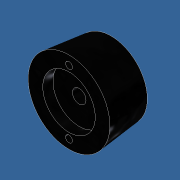
# Autodesk Inventor part: bouton
Saved by Autodesk Inventor 2015 SP2 (Build 190223200, 223)
## iProperties
Created: 2017-10-26
Part Number: bouton
Material: Générique
Document SubType Name: Modeling
Designer: Benoit.CURCHOD2
Density: 1 g/cm^3
Appearance: Noir
Author: Benoit.CURCHOD2
Autodesk Inventor part; units mm, degrees
ref_plane "YZ Plane" through (0, 0, 0) normal (1, 0, 0) x (0, 1, 0)
ref_plane "XZ Plane" through (0, 0, 0) normal (0, 1, 0) x (-1, 0, 0)
ref_plane "XY Plane" through (0, 0, 0) normal (0, 0, 1) x (1, 0, 0)
sketch "Esquisse1" plane through (0, 0, 0) normal (0, 0, 1) x (1, 0, 0)
  line L0 (-18, 0) -> (-16, 18.5)
  line L1 (-16, 18.5) -> (0, 18.5)
  line L2 (0, 15.5) -> (-3, 15.5)
  line L3 (-3, 15.5) -> (-3, 4.5)
  line L4 (-3, 4.5) -> (-11.55, 4.5)
  line L5 (-11.55, 4.5) -> (-11.55, 0)
  line L6 (-11.55, 0) -> (-18, 0)
  line L7 (0, -3.7) -> (0, 22.2) construction
  line L8 (-21.6, 0) -> (3.6, 0) construction
  line L9 (0, 18.5) -> (0, 15.5)
  point P0 (0, 0)
  dimension "d0" = 4.5
  dimension "d2" = 11
  dimension "d3" = 6
  dimension "d4" = 36
  dimension "d5" = 23.1
  dimension "d6" = 32
  dimension "d8" = 18.5
  constraints: 16 end point, 4 perpendicular, 2 collinear, 1 horizontal, 1 point on line
  measures "d0" distance between parallel lines of L8 L4
  measures "d2" distance between parallel lines of L4 L2
  measures "d3" diameter of L3 L7
  measures "d4" diameter of L0.start L7
  measures "d5" diameter of L5 L7
  measures "d6" diameter of L0.end L7
  measures "d8" distance between parallel lines of L1 L6
revolve "Révolution1" add sketch "Esquisse1" angle 360 about axis through (0, -10, 0) along (0, 1, 0)
sketch "Esquisse2" plane through (0, 0, 0) normal (0, -1, 0) x (1, 0, 0)
  circle A0 centre (0, 0) radius 14 construction
  circle A1 centre (0, -14) radius 1.5
  line L0 (0, -25.2) -> (0, 25.2) construction
  circle A2 centre (0, 14) radius 1.5
  dimension "d10" = 28
  dimension "d11" = 3
  dimension "d14" = 3
  constraints: 3 centre point, 2 point on circle, 2 point on line, 1 coincident
  measures "d10" diameter of A0
  measures "d11" diameter of A1
  measures "d14" diameter of A2
extrude "Extrusion1" cut sketch "Esquisse2" against normal blind 7
